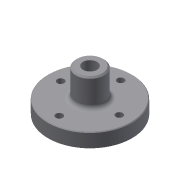
# Autodesk Inventor part: Flange
Saved by Autodesk Inventor 2022 (Build 260148000, 148)
## iProperties
Shininess: 64.0
Length Units: 11269
Angle Units: 11279
Time Units: 11290
Mass Units: 11283
Length Display Precision: 3
Angle Display Precision: 2
Compacted: True
Part Number: Flange
Document SubType Name: Modeling
Created: 2004-04-13
Designer: mpaknia
Manufacturer: Standard
Standards Organization: Custom
Density: 1 g/cm^3
Material: Generic
Appearance: Default
Density: 0.0
Volumn: 0.0
Area: 0.0
PropertySet Name: Model Information
Control State: 0
Master: False
Checked Out: False
Author: mpaknia
Autodesk Inventor part; units mm, degrees
ref_plane "YZ Plane" through (0, 0, 0) normal (1, 0, 0) x (0, 1, 0)
ref_plane "XZ Plane" through (0, 0, 0) normal (0, 1, 0) x (-1, 0, 0)
ref_plane "XY Plane" through (0, 0, 0) normal (0, 0, 1) x (1, 0, 0)
sketch "Sketch1" plane through (0, 0, 0) normal (0, 0, 1) x (1, 0, 0)
  circle A0 centre (0, 0) radius 30
  dimension "d0" = 60
  constraints: 1 centre point, 1 coincident
  measures "d0" diameter of A0
extrude "Extrusion1" add sketch "Sketch1" along normal mid plane 10
sketch "Sketch2" plane through (0, 0, 5) normal (0, 0, 1) x (1, 0, 0)
  circle A0 centre (0, 0) radius 30 projected
  circle A1 centre (0, 0) radius 10
  dimension "d3" = 20
  constraints: 1 centre point, 1 coincident
  measures "d3" diameter of A1
extrude "Extrusion2" add sketch "Sketch2" along normal blind 20 contours A1
sketch "Sketch3" plane through (0, 0, 25) normal (0, 0, 1) x (1, 0, 0)
  circle A0 centre (0, 0) radius 10 projected
  circle A1 centre (0, 0) radius 5
  dimension "d6" = 10
  constraints: 1 centre point, 1 coincident
  measures "d6" diameter of A1
extrude "Extrusion3" cut sketch "Sketch3" against normal through all contours A1
fillet "Fillet1" radius 3 1 edges at (-10, 0, 5)
chamfer "Chamfer1" distance 1 angle 45 1 edges at (-10, 0, 25)
sketch "Sketch5" plane through (0, 0, 5) normal (0, 0, 1) x (1, 0, 0)
  circle A0 centre (0, 0) radius 30 projected
  circle A1 centre (0, 0) radius 5 projected
  point P0 (-21, 0)
  point P1 (21, 0)
  point P2 (0, 22)
  point P3 (0, -22)
  dimension "d14" = 21
  dimension "d15" = 22
  dimension "d16" = 21
  dimension "d17" = 22
  constraints: 2 horizontal alignment, 2 vertical alignment
  measures "d14" distance of A1.centre point (-21, 0)
  measures "d15" distance of A0.centre point (0, 22)
  measures "d16" distance of A0.centre point (21, 0)
  measures "d17" distance of A0.centre point (0, -22)
hole "Hole1" at (-21, 0, 5) at (21, 0, 5) at (0, 22, 5) at (0, -22, 5) direction (0, 0, -1) diameter 5 end through all
chamfer "Chamfer2" distance 0.5 angle 45 1 edges at (-30, 0, 5)
body "Solid1"
